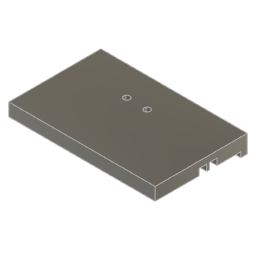
RedLigth_PCB_Shield (Autodesk Fusion 360 design; units mm, degrees)
Autodesk Fusion 360 part; units mm, degrees
sketch "Sketch1" plane through (0, 0, 0) normal (0, 0, 1) x (1, 0, 0)
  line L0 (20.3, 7.75) -> (-20.3, 7.75)
  line L1 (-20.3, 7.75) -> (-20.3, -7.75)
  line L2 (-20.3, -7.75) -> (20.3, -7.75)
  line L3 (20.3, -7.75) -> (20.3, 7.75)
  line L4 (20.3, 7.75) -> (-20.3, -7.75) construction
  line L5 (-20.3, 7.75) -> (20.3, -7.75) construction
  line L6 (17.8, 7.75) -> (17.8, -7.75) construction
  circle A0 centre (17.8, 2.35) radius 0.75
  circle A1 centre (17.8, 0.35) radius 0.75
  line L7 (-14.8, 7.75) -> (-14.8, -7.75)
  circle A2 centre (-14.8, -1.25) radius 0.75
  circle A3 centre (-14.8, 1.65) radius 0.75
  dimension "d1" = 40.6
  dimension "d2" = 15.5
  dimension "d5" = 2.5
  dimension "d6" = 1.5
  dimension "d7" = 5.4
  dimension "d8" = 1.5
  dimension "d9" = 2
  dimension "d10" = 5.5
  dimension "d11" = 6.5
  dimension "d12" = 6.1
  dimension "d13" = 1.5
  dimension "d14" = 1.5
  constraint horizontal L0
  constraint perpendicular L0 L1
  constraint parallel L0 L2
  constraint parallel L1 L3
  constraint coincident L4 origin
  constraint coincident L5 origin
  constraint coincident L0 L6.start
  constraint coincident L2 L6.end
  constraint perpendicular L2 L6
  constraint coincident L6 A0.centre
  constraint coincident L0 L7.start
  constraint coincident L2 L7.end
  constraint perpendicular L2 L7
  constraint coincident L7 A2.centre
  constraint coincident L7 A3.centre
  measures "d1" distance of L1.end L2.end
  measures "d2" distance of L0.end L1.end
  measures "d5" distance of L3 L6
  measures "d6" diameter of A0
  measures "d7" distance of L0 A0.centre
  measures "d8" diameter of A1
  measures "d9" distance of A0.centre A1.centre
  measures "d10" distance of L1 L7
  measures "d11" distance of L2 A2.centre
  measures "d12" distance of L0 A3.centre
  measures "d13" diameter of A3
  measures "d14" diameter of A2
extrude "Extrude1" add sketch "Sketch1" along normal blind 1 contours L0 L2 L3 L7 A2 A3 | L0 L1 L2 L7 A2 A3 makes body 1
sketch "Sketch1 (2)" plane through (0, 0, 1) normal (0, 0, 1) x (-1, 0, 0) in component "Plastique"
  circle A0 centre (-17.8, -2.35) radius 0.75
  circle A1 centre (14.8, 1.25) radius 0.75
  circle A2 centre (-17.8, -0.35) radius 0.75
  circle A3 centre (14.8, -1.65) radius 0.75
  line L0 (-20.3, 7.75) -> (-20.3, -7.75)
  line L1 (-20.3, -7.75) -> (20.3, -7.75)
  line L2 (20.3, -7.75) -> (20.3, 7.75)
  line L3 (20.3, 7.75) -> (-20.3, 7.75)
  line L4 (12.8, -7.75) -> (-15.8, -7.75)
  line L5 (-15.8, -7.75) -> (-15.8, 7.75)
  line L6 (-15.8, 7.75) -> (12.8, 7.75)
  line L7 (12.8, 7.75) -> (12.8, -7.75)
  line L8 (0, -7.75) -> (0, 7.75) construction
  line L9 (20.3, -3.25) -> (-15.8, -3.25) construction
  ellipse E0 centre (0, -3.25) end of major axis (-3, -3.25) minor radius 2.5
  line L10 (3, -3.25) -> (-3, -3.25)
  line L11 (0, -0.75) -> (0, -5.75)
  circle A4 centre (-2, -3.25) radius 0.6
  circle A5 centre (2, -3.25) radius 0.6
  line L12 (12.8, -2.4) -> (14.8, -2.4) construction
  line L13 (12.8, -0.9) -> (14.8, -0.9) construction
  line L14 (12.8, 0.5) -> (14.8, 0.5) construction
  line L15 (20.3, 0.5) -> (20.3, 2)
  line L16 (14.8, 2) -> (12.8, 2) construction
  line L17 (12.8, 2) -> (12.8, 0.5)
  line L18 (12.8, -2.4) -> (2.6, -2.4)
  line L19 (12.8, -0.9) -> (12.8, -2.4)
  line L20 (2.6, -3.25) -> (1.4, -3.25)
  line L21 (1.4, -3.25) -> (1.4, -0.9)
  line L22 (2.6, -2.4) -> (2.6, -3.25)
  line L23 (1.4, -0.9) -> (12.8, -0.9)
  line L24 (-2.6, 2) -> (12.8, 2)
  line L25 (12.8, 2) -> (12.8, 0.5)
  line L26 (-2.6, -3.25) -> (-2.6, 2)
  line L27 (-1.4, -3.25) -> (-1.4, 0.5)
  line L28 (12.8, 0.5) -> (-1.4, 0.5)
  line L29 (-13.3, -7.75) -> (-12.1, -7.75)
  line L30 (-12.1, -7.75) -> (-12.1, -1.6)
  line L31 (-12.1, -1.6) -> (-15.8, -1.6)
  line L32 (-13.3, -3.1) -> (-13.3, -7.75)
  line L33 (-10.1, -7.75) -> (-8.9, -7.75)
  line L34 (-8.9, -7.75) -> (-8.9, 0.4)
  line L35 (-10.1, -1.1) -> (-10.1, -7.75)
  line L36 (-15.8, -3.1) -> (-13.3, -3.1)
  line L37 (-8.9, 0.4) -> (-15.8, 0.4)
  line L38 (-15.8, -1.1) -> (-10.1, -1.1)
  ellipse E1 centre (0, -3.25) end of major axis (-4, -3.25) minor radius 3.6148
  line L39 (4, -3.25) -> (-4, -3.25)
  line L40 (0, 0.3648) -> (0, -6.8648)
  dimension "d18" = 2
  dimension "d19" = 2
  dimension "d39" = 20.3
  dimension "d40" = 11
  dimension "d41" = 5
  dimension "d42" = 1.2
  dimension "d43" = 1.2
  dimension "d44" = 1
  dimension "d45" = 1
  dimension "d46" = 1.2
  dimension "d47" = 1.2
  dimension "d48" = 7
  dimension "d49" = 1.2
  dimension "d50" = 2
  constraint horizontal L4
  constraint vertical L5
  constraint horizontal L6
  constraint vertical L7
  constraint coincident L3 L5.end
  constraint coincident L1 L4.start
  constraint coincident L4 L8.start
  constraint coincident L3 L8.end
  constraint perpendicular L6 L8
  constraint coincident L2 L9.start
  constraint perpendicular L0 L9
  constraint coincident E0 L10.start
  constraint coincident E0 L10.end
  constraint coincident E0 L11.start
  constraint coincident E0 L11.end
  constraint perpendicular L8 L10
  constraint coincident L9 A4.centre
  constraint coincident L9 A5.centre
  constraint coincident L7 L12.start
  constraint perpendicular L2 L12
  constraint tangent A3 L12
  constraint coincident L7 L13.start
  constraint perpendicular L2 L13
  constraint tangent A3 L13
  constraint horizontal L14
  constraint vertical L15
  constraint horizontal L16
  constraint vertical L17
  constraint coincident L2 L15.end
  constraint coincident L7 L14.start
  constraint tangent A1 L14
  constraint tangent A1 L16
  constraint coincident A3 L12.end
  constraint coincident A3 L13.end
  constraint coincident A1 L14.end
  constraint coincident A1 L16.start
  constraint horizontal L18
  constraint vertical L19
  constraint horizontal L20
  constraint vertical L21
  constraint vertical L22
  constraint coincident A5 L20.start
  constraint coincident L10 L20.start
  constraint perpendicular L19 L23
  constraint horizontal L28
  constraint horizontal L24
  constraint vertical L25
  constraint coincident L9 L26.start
  constraint coincident A4 L26.start
  constraint tangent A4 L26
  constraint coincident A4 L27.start
  constraint coincident L10 L27.start
  constraint tangent A4 L27
  constraint horizontal L29
  constraint vertical L30
  constraint horizontal L31
  constraint vertical L32
  constraint coincident L1 L29.start
  constraint horizontal L33
  constraint vertical L34
  constraint vertical L35
  constraint coincident L4 L33.start
  constraint tangent A0 L31
  constraint perpendicular L30 L36
  constraint tangent A0 L36
  constraint coincident L5 L36.start
  constraint coincident L5 L9.end
  constraint coincident L9 E0.centre
  constraint tangent A2 L37
  constraint tangent A2 L38
  constraint perpendicular L35 L38
  constraint coincident L5 L38.start
  constraint coincident L5 L37.end
  constraint coincident L5 L31.end
  constraint coincident E1 L39.start
  constraint coincident E1 L39.end
  constraint coincident E1 L40.start
  constraint coincident E1 L40.end
  constraint concentric E0 E1
  constraint parallel L9 L39
  measures "d18" distance of A0.centre L5
  measures "d19" distance of A3.centre L7
  measures "d39" distance of L2 L8
  measures "d40" distance of L3 L9
  measures "d42" diameter of A4
  measures "d43" diameter of A5
  measures "d44" distance of L10.end A4.centre
  measures "d45" distance of L10.start A5.centre
  measures "d46" distance of L20.start L20.end
  measures "d47" distance of L30 L32
  measures "d48" distance of L0 L32
  measures "d49" distance of L34 L35
  measures "d50" distance of L30 L35
extrude "Extrude1'" add sketch "Sketch1 (2)" along normal blind 2.5 separate body contours L1 L3 L4 L5 L6 L7 L18 L24 L26 L34 L37 E1 | L1 L4 L5 L32 L36 | L1 L4 L5 L33 L34 L35 L37 L38 | L1 L4 L5 L29 L30 L31 L32 L36 | L7 L17 L24 L25 L26 L27 L28 E1 | L1 L4 L5 L30 L31 L35 L38 | L7 L23 L27 L28 E1 | L7 L18 L19 L23 E1 | E0 L26 L27 E1 | E0 L26 E1 L39 | E0 L18 L21 L23 E1 | E0 L21 L23 E1 L40 | E0 L27 E1 L40 | E0 L10 L26 L39 | E0 A4 L26 L27 | E0 E1 L39 L40 | E0 L18 E1 L39 | E0 L10 L11 L27 L39 L40 | E0 L10 L11 A4 L39 L40 | L10 A4 L39 | L10 A4 L39 | E0 E1 L39 L40 | E0 A5 L18 L21 L22 | E0 L10 L18 L22 L39 | E0 L10 L11 L21 L39 L40 | E0 L10 L11 A5 L39 L40 | L10 A5 L20 L39 | L10 A5 L20 L39 makes body 2 in component "Plastique"
extrude "Extrude2" cut sketch "Sketch1 (2)" along normal blind 1.25 contours L1 L4 L5 L33 L34 L35 L37 L38 | L1 L4 L5 L29 L30 L31 L32 L36 | L7 L17 L24 L25 L26 L27 L28 E1 | L7 L18 L19 L23 E1 | E0 L26 L27 E1 | E0 L18 L21 L23 E1 | E0 A4 L26 L27 | L10 A4 L39 | L10 A4 L39 | E0 A5 L18 L21 L22 | L10 A5 L20 L39 | L10 A5 L20 L39 bodies 2 in component "Plastique"
extrude "Extrude3" cut sketch "Sketch1 (2)" along normal blind 2.5 contours L10 A4 L39 | L10 A4 L39 | L10 A5 L20 L39 | L10 A5 L20 L39 bodies 2 in component "Plastique"
sketch "Sketch2" plane through (0, 0, 3.5) normal (0, 0, 1) x (-1, 0, 0) in component "Plastique"
  circle A0 centre (2, -3.25) radius 0.6
  circle A1 centre (-2, -3.25) radius 0.6
  line L0 (-15.8, -7.75) -> (12.8, -7.75)
  line L1 (12.8, -7.75) -> (12.8, 7.75)
  line L2 (12.8, 7.75) -> (-15.8, 7.75)
  line L3 (-15.8, 7.75) -> (-15.8, -7.75)
  line L4 (20.3, -3.25) -> (-15.8, -3.25)
  line L5 (0, -7.75) -> (0, 7.75)
  ellipse E0 centre (0, -3.25) end of major axis (4, -3.25) minor radius 3.5
  line L6 (-4, -3.25) -> (4, -3.25)
  line L7 (0, -6.75) -> (0, 0.25)
  ellipse E1 centre (0, -3.25) end of major axis (3, -3.25) minor radius 2.5
  line L8 (-3, -3.25) -> (3, -3.25)
  line L9 (0, -5.75) -> (0, -0.75)
  dimension "d58" = 7
  dimension "d59" = 5
  constraint coincident E0 L6.start
  constraint coincident E0 L6.end
  constraint coincident E0 L7.start
  constraint coincident E0 L7.end
  constraint coincident L5 E0.centre
  constraint coincident L4 E0.centre
  constraint perpendicular L5 L6
  constraint coincident E1 L8.start
  constraint coincident E1 L8.end
  constraint coincident E1 L9.start
  constraint coincident E1 L9.end
  constraint concentric E0 E1
  constraint perpendicular L7 L8
extrude "Extrude4" add sketch "Sketch2" along normal blind 1 contours A0 L4 L5 L6 L7 E1 L8 L9 | A0 L4 L5 L6 L7 E1 L8 L9 | L4 L5 E0 L6 L7 E1 | L4 L5 E0 L6 L7 E1 | A1 L4 L5 L6 L7 E1 L8 L9 | A1 L4 L5 L6 L7 E1 L8 L9 | L4 L5 E0 L6 L7 E1 | L4 L5 E0 L6 L7 E1 bodies 2 in component "Plastique"
extrude "Extrude5" add sketch "Sketch2" along normal blind 2 contours L4 L5 E0 L6 L7 E1 | L4 L5 E0 L6 L7 E1 | L4 L5 E0 L6 L7 E1 | L4 L5 E0 L6 L7 E1 bodies 2 in component "Plastique"
extrude "Extrude6" add 1 faces at (-5.5667, 7.75, 2.25) along direction (0, 1, 0) blind 1.25 on bodies 2 bodies 2 in component "Plastique"
extrude "Extrude7" add 1 faces at (-3.2667, -7.75, 2.6667) along direction (0, -1, 0) blind 1.25 on bodies 2 bodies 2 in component "Plastique"
sketch "Sketch3" plane through (0, 0, 1) normal (0, 0, -1) x (1, 0, 0) in component "Plastique"
  line L0 (-2.6, -2.4) -> (-12.8, -2.4)
  line L1 (-12.8, -2.4) -> (-12.8, -9)
  line L2 (-12.8, -9) -> (8.9, -9)
  line L3 (8.9, -9) -> (8.9, 0.4)
  line L4 (8.9, 0.4) -> (15.8, 0.4)
  line L5 (15.8, 0.4) -> (15.8, 9)
  line L6 (15.8, 9) -> (-12.8, 9)
  line L7 (-12.8, 9) -> (-12.8, 2)
  line L8 (-12.8, 2) -> (2.6, 2)
  line L9 (2.6, 2) -> (2.6, -3.25)
  arc A0 (1.4, -3.25) -> (2.6, -3.25) centre (2, -3.25) ccw
  line L10 (1.4, -3.25) -> (1.4, 0.5)
  line L11 (1.4, 0.5) -> (-12.8, 0.5)
  line L12 (-12.8, 0.5) -> (-12.8, -0.9)
  line L13 (-12.8, -0.9) -> (-1.4, -0.9)
  line L14 (-1.4, -0.9) -> (-1.4, -3.25)
  arc A1 (-2.6, -3.25) -> (-1.4, -3.25) centre (-2, -3.25) ccw
  line L15 (-2.6, -3.25) -> (-2.6, -2.4)
  circle A2 centre (17.8, -2.35) radius 0.75
  circle A3 centre (-14.8, 1.25) radius 0.75
  circle A4 centre (17.8, -0.35) radius 0.75
  circle A5 centre (-14.8, -1.65) radius 0.75
  line L16 (20.3, -7.75) -> (20.3, 7.75)
  line L17 (20.3, 7.75) -> (-20.3, 7.75)
  line L18 (-20.3, 7.75) -> (-20.3, -7.75)
  line L19 (-20.3, -7.75) -> (20.3, -7.75)
  line L20 (15.8, -1.1) -> (10.1, -1.1)
  line L21 (10.1, -1.1) -> (10.1, -9)
  line L22 (10.1, -9) -> (12.1, -9)
  line L23 (12.1, -9) -> (12.1, -1.6)
  line L24 (12.1, -1.6) -> (15.8, -1.6)
  line L25 (15.8, -1.6) -> (15.8, -1.1)
  line L26 (15.8, -3.1) -> (13.3, -3.1)
  line L27 (13.3, -3.1) -> (13.3, -9)
  line L28 (13.3, -9) -> (15.8, -9)
  line L29 (15.8, -9) -> (15.8, -3.1)
extrude "Extrude8" add sketch "Sketch3" along normal blind 2 contours L1 L2 L3 L19 | L19 L21 L22 L23 | L5 L6 L7 L17 | L19 L27 L28 L29 bodies 2 in component "Plastique"
sketch "Sketch4" plane through (0, 7.75, 0) normal (0, -1, 0) x (1, 0, 0) in component "Plastique"
  line L0 (15.8, 1) -> (13.3, 1)
  line L1 (13.3, 1) -> (13.3, -1)
  line L2 (13.3, -1) -> (15.8, -1)
  line L3 (15.8, -1) -> (15.8, 1)
  line L4 (17.05, 0) -> (18.55, 0)
  line L5 (-15.55, 0) -> (-14.05, 0)
  line L6 (17.05, 0) -> (18.55, 0)
  line L7 (-15.55, 0) -> (-14.05, 0)
  line L8 (20.3, 0) -> (-20.3, 0)
  line L9 (-20.3, 0) -> (20.3, 0)
  line L10 (12.1, 1) -> (10.1, 1)
  line L11 (10.1, 1) -> (10.1, -1)
  line L12 (10.1, -1) -> (12.1, -1)
  line L13 (12.1, -1) -> (12.1, 1)
  line L14 (8.9, 1) -> (-12.8, 1)
  line L15 (-12.8, 1) -> (-12.8, -1)
  line L16 (-12.8, -1) -> (8.9, -1)
  line L17 (8.9, -1) -> (8.9, 1)
extrude "Extrude9" add sketch "Sketch4" along normal blind 1.5 contours L1 L2 L3 L8 L9 | L8 L9 L11 L12 L13 | L8 L9 L15 L16 L17 bodies 2 in component "Plastique"
extrude "Extrude10" cut 2 faces at (14.1333, 6.25, -0.6667) (10.7667, 6.25, -0.3333) along direction (0, 1, 0) blind 4.5 on bodies 2 bodies 2 in component "Plastique"
sketch "Sketch5" plane through (0, -7.75, 0) normal (0, 1, 0) x (-1, 0, 0) in component "Plastique"
  line L0 (12.8, 1) -> (-15.8, 1)
  line L1 (-15.8, 1) -> (-15.8, -1)
  line L2 (-15.8, -1) -> (12.8, -1)
  line L3 (12.8, -1) -> (12.8, 1)
  line L4 (-18.55, 0) -> (-17.05, 0)
  line L5 (14.05, 0) -> (15.55, 0)
  line L6 (-18.55, 0) -> (-17.05, 0)
  line L7 (14.05, 0) -> (15.55, 0)
  line L8 (-20.3, 0) -> (20.3, 0)
  line L9 (20.3, 0) -> (-20.3, 0)
extrude "Extrude11" add sketch "Sketch5" along normal blind 2 contours L1 L2 L3 L8 L9 bodies 2 in component "Plastique"
sketch "Sketch2 (2)" plane through (0, 0, 0) normal (0, 0, 1) x (1, 0, 0) in component "Button"
  line L0 (-2, 2) -> (-2, -2)
  line L1 (-2, -2) -> (2, -2)
  line L2 (2, -2) -> (2, 2)
  line L3 (2, 2) -> (-2, 2)
  line L4 (1, 1.5) -> (1, -1.5)
  line L5 (1, -1.5) -> (-1, -1.5)
  line L6 (-1, -1.5) -> (-1, 1.5)
  line L7 (-1, 1.5) -> (1, 1.5)
  circle A0 centre (0, 0) radius 3
  circle A1 centre (0, 0) radius 2.375
  circle A2 centre (0, 0) radius 3.75
  dimension "d79" = 6
  dimension "d80" = 4.75
  dimension "d81" = 7.5
  constraint coincident A0.centre A1.centre
  constraint concentric A0 A2
  measures "d79" diameter of A0
  measures "d80" diameter of A1
  measures "d81" diameter of A2
extrude "Extrude1''" add sketch "Sketch2 (2)" against normal blind 1.8 separate body contours A0 makes body 3 in component "Button"
extrude "Extrude2'" add sketch "Sketch2 (2)" along normal blind 1.5 contours L0 L3 A1 | L0 L1 A1 | L2 L3 A1 | L1 L2 A1 | A0 | A2 bodies 3 in component "Button"
sketch "Sketch3 (2)" plane through (0, 0, 0) normal (0, 0, 1) x (1, 0, 0) in component "Button"
  circle A0 centre (0, 0) radius 2.125
  line L0 (1, -1.5) -> (-1, -1.5)
  line L1 (-1, -1.5) -> (-1, 1.5)
  line L2 (1, 1.5) -> (1, -1.5)
  line L3 (-1, 1.5) -> (1, 1.5)
  dimension "d87" = 4.25
  constraint coincident A0.centre origin
  measures "d87" diameter of A0
extrude "Extrude1'''" add sketch "Sketch3 (2)" along normal blind 3.5 separate body makes body 4 in component "Component'"
extrude "Extrude2''" add 1 faces at (-1.375, 0, 3.5) along direction (0, 0, 1) blind 1.5 separate body on bodies 4 makes body 5 in component "Component'"
extrude "Extrude3'" add 1 faces at (-0.3333, -1.5, 4.5) along direction (0, 1, 0) blind 3 on bodies 5 bodies 5 4 in component "Component'"
fillet "Fillet1" radius 0.5 1 edges at (-1.9812, -0.7684, 5) on bodies 5 in component "Component'"
extrude "Extrude4'" cut 1 faces at (-1.375, 0, 0) along direction (0, 0, 1) blind 0.5 on bodies 5 bodies 5 in component "Component'"
extrude "Extrude12" cut 1 faces at (6.2667, -7.0833, 0) along direction (0, 0, -1) blind 0.3 on bodies 2 bodies 2 in component "Plastique"
extrude "Extrude13" cut 1 faces at (1.6667, 6.75, 0) along direction (0, 0, -1) blind 0.3 on bodies 2 bodies 2 in component "Plastique"
extrude "Extrude14" add 2 faces at (6.2667, -6.8333, -1) (-5.5667, 7.1667, -1) along direction (0, 0, -1) blind 0.3 on bodies 2 bodies 2 in component "Plastique"
extrude "Extrude15" cut 1 faces at (0.2147, 0.0986, 5.5) along direction (0, 0, -1) blind 2 on bodies 2 bodies 2 in component "Plastique"
extrude "Extrude16" cut 1 faces at (0, 4.2569, 4.5) along direction (0, 0, -1) blind 1 on bodies 2 bodies 2 in component "Plastique"
extrude "Extrude1''''" add sketch "Sketch2" along normal blind 1 separate body contours A0 L4 L5 L6 L7 E1 L8 L9 | A0 L4 L5 L6 L7 E1 L8 L9 | L4 L5 E0 L6 L7 E1 | L4 L5 E0 L6 L7 E1 | A1 L4 L5 L6 L7 E1 L8 L9 | A1 L4 L5 L6 L7 E1 L8 L9 | L4 L5 E0 L6 L7 E1 | L4 L5 E0 L6 L7 E1 makes body 6 in component "Component''"
extrude "Extrude2'''" add sketch "Sketch2" along normal blind 2.5 contours L4 L5 E0 L6 L7 E1 | L4 L5 E0 L6 L7 E1 | L4 L5 E0 L6 L7 E1 | L4 L5 E0 L6 L7 E1 bodies 6 in component "Component''"
extrude "Extrusion17" cut 1 faces at (6.2667, -6.8333, -1.3) along direction (0, 0, 1) blind 2.3 on bodies 2 bodies 2 in component "Plastique"
extrude "Extrusion18" cut 1 faces at (-5.5667, 7.1667, -1.3) along direction (0, 0, 1) blind 2.3 on bodies 2 bodies 2 in component "Plastique"
component "Plastique" placed x (1, 0, 0) y (0, 1, 0) z (0, 0, 1) at (0, 0, 0)
component "Button" placed x (1, 0, 0) y (0, 1, 0) z (0, 0, 1) at (0, 0, 0)
component "Component''" placed x (1, 0, 0) y (0, 1, 0) z (0, 0, 1) at (0, 0, 0) in component "Plastique"
component "Component'" placed x (1, 0, 0) y (0, 1, 0) z (0, 0, 1) at (0, 0, 0) in component "Button"
hidden bodies 1
equation "d1 = wPcb"
equation "d2 = hPcb"
equation "hPcb = 15.5 mm"
equation "wPcb = 40.6 mm"
equation "d6 = d13"
equation "d8 = d13"
equation "d14 = d13"
equation "tPcb = 1 mm"
equation "d16 = tPcb"
equation "d39 = wPcb / 2"
equation "d49 = d47"
equation "tP = 2.5 mm"
equation "d52 = tP"
equation "d56 = tP"
equation "hPButton = 1.8 mm" comment "Hauteur du plastique"
equation "d83 = -hPButton"
named bodies: "PCB"
